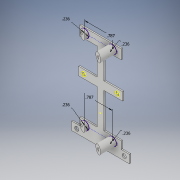
# Autodesk Inventor part: PI Rfid baracke angledt
Saved by Autodesk Inventor 2018 (Build 220112000, 112)
## iProperties
Created: 2019-09-27
Part Number: PI Rfid baracke angledt
Material: Generic
Document SubType Name: Modeling
Designer: Jacob
Density: 1 g/cm^3
Appearance: Default
Author: Jacob
Autodesk Inventor part; units mm, degrees
ref_plane "YZ Plane" through (0, 0, 0) normal (1, 0, 0) x (0, 1, 0)
ref_plane "XZ Plane" through (0, 0, 0) normal (0, 1, 0) x (-1, 0, 0)
ref_plane "XY Plane" through (0, 0, 0) normal (0, 0, 1) x (1, 0, 0)
sketch "Sketch1" plane through (0, 0, 0) normal (0, 0, 1) x (1, 0, 0)
  line L0 (-2.5, 15.5) -> (2.5, 15.5)
  line L1 (2.5, 15.5) -> (2.5, -15.5)
  line L2 (2.5, -15.5) -> (-2.5, -15.5)
  line L3 (-2.5, -15.5) -> (-2.5, 15.5)
  line L4 (-2.5, 15.5) -> (2.5, -15.5) construction
  line L5 (2.5, 15.5) -> (-2.5, -15.5) construction
  line L6 (0, 0) -> (0, 29.5852) construction
  line L7 (-16, 21.5) -> (16, 21.5)
  line L8 (16, 21.5) -> (16, 15.5)
  line L9 (16, 15.5) -> (-16, 15.5)
  line L10 (-16, 15.5) -> (-16, 21.5)
  line L11 (-16, 21.5) -> (16, 15.5) construction
  line L12 (16, 21.5) -> (-16, 15.5) construction
  line L13 (0, 0) -> (0, -27.9929) construction
  line L14 (-21, -15.5) -> (21, -15.5)
  line L15 (21, -15.5) -> (21, -21.5)
  line L16 (21, -21.5) -> (-21, -21.5)
  line L17 (-21, -21.5) -> (-21, -15.5)
  line L18 (-21, -15.5) -> (21, -21.5) construction
  line L19 (21, -15.5) -> (-21, -21.5) construction
  line L20 (16, 18.5) -> (-16, 18.5) construction
  line L21 (21, -18.5) -> (-21, -18.5) construction
  point P0 (0, 18.5)
  point P1 (0, -18.5)
  dimension "d0" = 5
  dimension "d2" = 32
  dimension "d3" = 6
  dimension "d4" = 0
  dimension "d5" = 42
  dimension "d6" = 6
  dimension "d7" = 0
  dimension "d65" = 37
  constraints: 44 end point, 10 midpoint, 7 parallel, 3 horizontal, 3 perpendicular, 2 point on line, 1 vertical
  measures "d0" distance between parallel lines of L1 L3
  measures "d2" distance of L7.start L7.end
  measures "d3" distance of L7.end L8.end
  measures "d4" distance between parallel lines of L0 L9
  measures "d5" distance of L15.end L16.end
  measures "d6" distance of L14.end L15.end
  measures "d7" distance between parallel lines of L2 L14
  measures "d65" vertical distance of L21.start L20.start
extrude "Extrusion1" add sketch "Sketch1" along normal blind 1
sketch "Sketch2" plane through (0, 0, 1) normal (0, 0, 1) x (1, 0, 0)
  line L0 (-16, 21.5) -> (-16, 15.5) projected
  line L1 (-16, 18.5) -> (16, 18.5) construction
  line L2 (16, 15.5) -> (16, 21.5) projected
  line L3 (-21, -15.5) -> (-21, -21.5) projected
  line L4 (-21, -18.5) -> (21, -18.5) construction
  line L5 (21, -15.5) -> (21, -21.5) projected
  circle A0 centre (-17.25, -18.5) radius 1.5
  circle A1 centre (17.25, -18.5) radius 1.5
  line L6 (0, 0) -> (0, -21.5) construction
  line L7 (21, -21.5) -> (-21, -21.5) projected
  line L8 (0, 0) -> (0, 21.5) construction
  line L9 (16, 21.5) -> (-16, 21.5) projected
  circle A2 centre (-12.25, 18.5) radius 1.5
  circle A3 centre (12.25, 18.5) radius 1.5
  dimension "d10" = 34.5
  dimension "d13" = 17.25
  dimension "d14" = 17.25
  dimension "d15" = 3
  dimension "d16" = 3
  dimension "d17" = 24.5
  dimension "d18" = 12.25
  dimension "d19" = 12.25
  dimension "d20" = 3
  dimension "d21" = 3
  dimension "d66" = 37
  constraints: 8 end point, 6 midpoint, 4 centre point, 4 point on line
  measures "d10" distance of A1.centre A0.centre
  measures "d13" distance from line of L6 A0.centre
  measures "d14" distance from line of L6 A1.centre
  measures "d15" diameter of A0
  measures "d16" diameter of A1
  measures "d17" distance of A3.centre A2.centre
  measures "d18" distance from line of L8 A2.centre
  measures "d19" distance from line of L8 A3.centre
  measures "d20" diameter of A2
  measures "d21" diameter of A3
  measures "d66" distance between parallel lines of L4 L1
extrude "Extrusion2" cut sketch "Sketch2" against normal blind 2
sketch "Sketch4" plane through (0, 0, 1) normal (0, 0, 1) x (1, 0, 0)
  line L0 (0, 0) -> (0, 68.1033) construction
  line L1 (0, 0) -> (0, -40.1743) construction
  line L2 (-15, 48) -> (15, 48)
  line L3 (15, 48) -> (15, 41)
  line L4 (15, 41) -> (-15, 41)
  line L5 (-15, 41) -> (-15, 48)
  line L6 (-15, 48) -> (15, 41) construction
  line L7 (15, 48) -> (-15, 41) construction
  line L8 (-15, -10) -> (15, -10)
  line L9 (15, -10) -> (15, -17)
  line L10 (15, -17) -> (-15, -17)
  line L11 (-15, -17) -> (-15, -10)
  line L12 (-15, -10) -> (15, -17) construction
  line L13 (15, -10) -> (-15, -17) construction
  circle A0 centre (-17.25, -18.5) radius 1.5 projected
  line L14 (-2.5, 41) -> (2.5, 41)
  line L15 (2.5, 41) -> (2.5, 21.5)
  line L16 (2.5, 21.5) -> (-2.5, 21.5)
  line L17 (-2.5, 21.5) -> (-2.5, 41)
  line L18 (-2.5, 41) -> (2.5, 21.5) construction
  line L19 (2.5, 41) -> (-2.5, 21.5) construction
  line L20 (16, 21.5) -> (-16, 21.5) projected
  line L21 (-15, -13.5) -> (15, -13.5) construction
  line L22 (-15, 44.5) -> (15, 44.5) construction
  circle A1 centre (-11.5, -13.5) radius 1
  circle A2 centre (11.5, -13.5) radius 1
  circle A3 centre (-11.5, 44.5) radius 1
  circle A4 centre (11.5, 44.5) radius 1
  point P0 (0, 44.5)
  point P1 (0, -13.5)
  point P2 (0, 31.25)
  dimension "d28" = 58
  dimension "d29" = 5
  dimension "d30" = 0
  dimension "d31" = 0
  dimension "d32" = 5
  dimension "d33" = 30
  dimension "d34" = 30
  dimension "d35" = 7
  dimension "d36" = 7
  dimension "d37" = 2
  dimension "d38" = 2
  dimension "d39" = 2
  dimension "d40" = 2
  dimension "d41" = 23
  dimension "d42" = 23
  dimension "d43" = 11.5
  dimension "d44" = 11.5
  dimension "d45" = 11.5
  dimension "d46" = 11.5
  constraints: 44 end point, 10 midpoint, 7 point on line, 6 parallel, 4 centre point, 3 horizontal, 3 perpendicular, 2 vertical
  measures "d28" distance of point (0, -13.5) point (0, 44.5)
  measures "d29" vertical distance of A0.centre point (0, -13.5)
  measures "d30" distance between parallel lines of L20 L16
  measures "d31" distance between parallel lines of L4 L14
  measures "d32" distance between parallel lines of L15 L17
  measures "d33" distance between parallel lines of L9 L11
  measures "d34" distance between parallel lines of L3 L5
  measures "d35" distance of L2.end L3.end
  measures "d36" distance of L8.end L9.end
  measures "d37" diameter of A3
  measures "d38" diameter of A4
  measures "d39" diameter of A1
  measures "d40" diameter of A2
  measures "d41" distance of A2.centre A1.centre
  measures "d42" distance of A4.centre A3.centre
  measures "d43" distance from line of L0 A3.centre
  measures "d44" distance from line of L0 A4.centre
  measures "d45" distance from line of L1 A1.centre
  measures "d46" distance from line of L1 A2.centre
extrude "Extrusion3" add sketch "Sketch4" against normal blind 1 contours L2 L3 L4 L5 | L4 L15 L16 L17 | L8 L9 L10 L11
sketch "Sketch5" plane through (0, 0, 1) normal (0, 0, 1) x (1, 0, 0)
  circle A0 centre (-12.25, 18.5) radius 1.5 projected
  circle A1 centre (12.25, 18.5) radius 1.5 projected
  circle A2 centre (-11.5, -13.5) radius 3
  circle A3 centre (-11.5, 44.5) radius 3
  line L0 (-11.5, -13.5) -> (11.5, -13.5) construction
  circle A4 centre (8.5, -13.5) radius 3
  circle A5 centre (-11.5, 44.5) radius 1 projected
  line L1 (-11.5, 44.5) -> (11.5, 44.5) construction
  circle A6 centre (8.5, 44.5) radius 3
  point P0 (0, 0)
  dimension "d52" = 6
  dimension "d55" = 6
  dimension "d97" = 6
  dimension "d98" = 20
  dimension "d99" = 6
  dimension "d100" = 20
  constraints: 4 centre point, 4 end point, 2 coincident, 2 horizontal, 2 point on line
  measures "d52" diameter of A2
  measures "d55" diameter of A3
  measures "d97" diameter of A4
  measures "d98" distance of A4.centre A2.centre
  measures "d99" diameter of A6
  measures "d100" distance of A6.centre A3.centre
extrude "Extrusion5" [suppressed]
sketch "Sketch6" plane through (0, 0, 0) normal (0, 0, -1) x (-1, 0, 0)
  circle A0 centre (-17.25, -18.5) radius 1.5 projected
  circle A1 centre (-17.25, -18.5) radius 3
  circle A2 centre (17.25, -18.5) radius 1.5 projected
  circle A3 centre (17.25, -18.5) radius 3
  circle A4 centre (12.25, 18.5) radius 1.5 projected
  circle A5 centre (12.25, 18.5) radius 3
  circle A6 centre (-12.25, 18.5) radius 1.5 projected
  circle A7 centre (-12.25, 18.5) radius 3
  point P0 (0, 0)
  dimension "d59" = 6
  dimension "d60" = 6
  dimension "d61" = 6
  dimension "d62" = 6
  constraints: 4 centre point, 4 coincident
  measures "d59" diameter of A7
  measures "d60" diameter of A5
  measures "d61" diameter of A1
  measures "d62" diameter of A3
extrude "Extrusion6" [suppressed]
sketch "Sketch8" plane through (-21, -21.5, 0) normal (0, -1, 0) x (1, 0, 0)
  line L0 (35.5, 13.7) -> (29.5, 13.7) construction
  line L1 (35.5, 1) -> (35.5, 13.7) construction
  line L2 (29.5, 1) -> (29.5, 13.7) construction
  line L3 (6.5, 1) -> (6.5, 7.35) construction
  line L4 (12.5, 7.35) -> (6.5, 7.35) construction
  line L5 (12.5, 1) -> (12.5, 7.35) construction
  line L6 (0, 1) -> (42, 1) construction
  line L7 (35.5, 13.7) -> (6.5, 1.3902)
  line L8 (35.5, 13.7) -> (6.5, 13.7)
  line L9 (6.5, 13.7) -> (6.5, 1.3902)
  point P0 (21, 0)
  dimension "d72" = 67
  constraints: 6 end point, 1 collinear, 1 horizontal, 1 point on line
  measures "d72" angle of L1 L7
extrude "Extrusion9" add sketch "Sketch5" along normal blind 6.35 contours A2 | A3 | A5
extrude "Extrusion14" add sketch "Sketch5" along normal blind 12 contours A4 | A6
extrude "Extrusion11" cut sketch "Sketch8" against normal blind 76.2
sketch "Sketch9" plane through (-11.5, -13.5, 2.6637) normal (-0.3907311, 0, 0.9205049) x (0.9205049, 0, 0.3907311)
  line L0 (7.2438, 54.5) -> (-4.2625, 54.5) projected
  line L1 (28.8393, 61.5) -> (-3.7762, 61.5)
  line L2 (-3.7762, 61.5) -> (-3.7762, 54.5)
  line L3 (-3.7762, 54.5) -> (28.8393, 54.5)
  line L4 (28.8393, 54.5) -> (28.8393, 61.5)
  line L5 (28.8393, 3.5) -> (-3.7762, 3.5)
  line L6 (-3.7762, 3.5) -> (-3.7762, -3.0673)
  line L7 (-3.7762, -3.0673) -> (28.8393, -3.0673)
  line L8 (28.8393, -3.0673) -> (28.8393, 3.5)
  point P0 (9.545, 13.5)
  point P1 (-3.7762, -2)
  constraints: 16 end point, 4 parallel, 3 point on line, 2 horizontal, 2 perpendicular
extrude "Extrusion12" [suppressed]
sketch "Sketch10" plane through (-11.8907, -13.5, 3.5842) normal (-0.3907311, 0, 0.9205049) x (0.9205049, 0, 0.3907311)
  line L0 (24.0316, 58.2163) -> (1.0316, 58.2163) construction
  line L1 (1.0316, 58.2163) -> (1.0316, 0.2163) construction
  line L2 (1.0316, 0.2163) -> (24.0316, 0.2163) construction
  line L3 (24.0316, 0.2163) -> (24.0316, 58.2163) construction
  line L4 (-3.7762, -3.0673) -> (28.8393, -3.0673) projected
  line L5 (28.8393, 61.5) -> (-3.7762, 61.5) projected
  line L6 (28.8393, 54.5) -> (28.8393, 61.5) projected
  line L7 (-3.7762, 61.5) -> (-3.7762, 54.5) projected
  circle A0 centre (24.0316, 58.2163) radius 1
  circle A1 centre (1.0316, 58.2163) radius 1
  circle A2 centre (1.0316, 0.2163) radius 1
  circle A3 centre (24.0316, 0.2163) radius 1
  point P0 (9.545, 13.5)
  dimension "d81" = 23
  dimension "d82" = 58
  dimension "d83" = 3.2837
  dimension "d84" = 3.2837
  dimension "d85" = 4.8078
  dimension "d86" = 4.8078
  dimension "d87" = 2
  dimension "d88" = 2
  dimension "d89" = 2
  dimension "d90" = 2
  constraints: 8 end point, 4 centre point, 4 coincident, 2 parallel, 1 horizontal, 1 perpendicular
  measures "d81" distance of L0.start L0.end
  measures "d82" distance of L2.end L0.start
  measures "d83" distance between parallel lines of L4 L2
  measures "d84" distance between parallel lines of L5 L0
  measures "d85" distance between parallel lines of L3 L6
  measures "d86" distance between parallel lines of L7 L1
  measures "d87" diameter of A3
  measures "d88" diameter of A2
  measures "d89" diameter of A0
  measures "d90" diameter of A1
extrude "Extrusion13" [suppressed]
sketch "Sketch12" plane through (-11.5, -13.5, 2.6637) normal (-0.3907311, 0, 0.9205049) x (0.9205049, 0, 0.3907311)
  ellipse E0 centre (21.7272, 0) end of major axis (18.4681, 0) minor radius 3 projected
  ellipse E1 centre (0, 0) end of major axis (-3.2591, 0) minor radius 3 projected
  ellipse E2 centre (21.7272, 58) end of major axis (18.4681, 58) minor radius 3 projected
  ellipse E3 centre (0, 58) end of major axis (-3.2591, 58) minor radius 3 projected
  line L0 (-3.2591, 0) -> (24.9863, 0) construction
  circle A0 centre (21.7909, 0) radius 1
  circle A1 centre (-1.2591, 0) radius 1
  line L1 (24.9863, 58) -> (-3.2591, 58) construction
  circle A2 centre (-1.2591, 58) radius 1
  circle A3 centre (21.7909, 58) radius 1
  point P0 (9.545, 13.5)
  dimension "d103" = 2
  dimension "d104" = 2
  dimension "d105" = 23.05
  dimension "d106" = 2
  dimension "d110" = 2
  dimension "d111" = 2
  dimension "d112" = 23.05
  dimension "d113" = 2
  constraints: 4 centre point, 4 end point, 4 horizontal alignment, 4 point on line, 2 horizontal, 4 other
  measures "d103" diameter of A0
  measures "d104" diameter of A1
  measures "d105" distance of A1.centre A0.centre
  measures "d106" distance of L0.start A1.centre
  measures "d110" diameter of A3
  measures "d111" diameter of A2
  measures "d112" distance of A3.centre A2.centre
  measures "d113" distance of L1.end A2.centre
extrude "Extrusion15" cut sketch "Sketch12" against normal blind 5 contours A0 | A1 | A2 | A3
equation "\"d13\" = d14"
equation "\"d18\" = d19"
equation "\"d43\" = d44"
equation "\"d45\" = d46"
equation "\"d83\" = d84"
equation "\"d85\" = d86"
body "Solid1"
